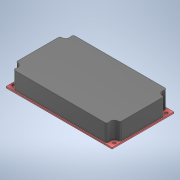
# Autodesk Inventor part: SUSTAINA-Core-Board
Saved by Autodesk Inventor 2022.3 (Build 263350000, 350)
## iProperties
Part Number: SUSTAINA-Core-Board
Material: 一般
Document SubType Name: Modeling
Designer: Masato Kubotera
Density: 1 g/cm^3
Appearance: 既定
Description: CircuitBoard
Author: Masato Kubotera
Autodesk Inventor part; units mm, degrees
ref_plane "YZ Plane" through (0, 0, 0) normal (1, 0, 0) x (0, 1, 0)
ref_plane "XZ Plane" through (0, 0, 0) normal (0, 1, 0) x (-1, 0, 0)
ref_plane "XY Plane" through (0, 0, 0) normal (0, 0, 1) x (1, 0, 0)
derived "Cockpit_circuit_board_frame.ipt"
sketch "スケッチ3" plane through (0, 0, -88.5) normal (0, 0, 1) x (1, 0, 0)
  line L0 (20.25, -135) -> (20.25, 0)
  line L1 (-83.25, 0) -> (-83.25, -135)
  line L2 (-31.5, -135) -> (-31.5, 0) construction
  line L3 (-83.25, -67.5) -> (20.25, -67.5) construction
  line L4 (-52.45, 1.4849) -> (-52.45, 5)
  line L5 (-52.45, 5) -> (-10.55, 5)
  line L6 (-10.55, 5) -> (-10.55, 1.4849)
  arc A0 (-53.9349, 0) -> (-52.45, 1.4849) centre (-53.1925, 0.7425) ccw
  arc A1 (-10.55, 1.4849) -> (-9.0651, 0) centre (-9.8075, 0.7425) ccw
  line L7 (-53.9349, 0) -> (-83.25, 0)
  line L8 (20.25, 0) -> (-9.0651, 0)
  line L9 (-10.55, 0) -> (-52.45, 0)
  line L10 (-10.55, -135) -> (-52.45, -135)
  arc A2 (-52.45, -136.4849) -> (-53.9349, -135) centre (-53.1925, -135.7425) ccw
  line L11 (-52.45, -136.4849) -> (-52.45, -140)
  line L12 (-52.45, -140) -> (-10.55, -140)
  line L13 (-10.55, -140) -> (-10.55, -136.4849)
  arc A3 (-9.0651, -135) -> (-10.55, -136.4849) centre (-9.8075, -135.7425) ccw
  line L14 (20.25, -135) -> (-9.0651, -135)
  line L15 (-53.9349, -135) -> (-83.25, -135)
  line L16 (18, -127.5) -> (-52, -127.5) construction
  line L17 (-52, -127.5) -> (-52, -7.5) construction
  line L18 (-52, -7.5) -> (18, -7.5) construction
  line L19 (18, -7.5) -> (18, -127.5) construction
  line L20 (18, -127.5) -> (-52, -7.5) construction
  line L21 (-52, -127.5) -> (18, -7.5) construction
  line L22 (-48.5, -116.5) -> (-48.5, -18.5)
  line L23 (-38.5627, -9.5) -> (4.5627, -9.5)
  line L24 (12.5, -10.5) -> (-46.5, -10.5) construction
  line L25 (-46.5, -10.5) -> (-46.5, -124.5) construction
  line L26 (-46.5, -124.5) -> (12.5, -124.5) construction
  line L27 (12.5, -124.5) -> (12.5, -10.5) construction
  line L28 (12.5, -10.5) -> (-46.5, -124.5) construction
  line L29 (-46.5, -10.5) -> (12.5, -124.5) construction
  circle A4 centre (12.5, -10.5) radius 2
  circle A5 centre (-46.5, -10.5) radius 2
  arc A6 (-46.5, -16.5) -> (-40.5471, -11.25) centre (-46.5, -10.5) ccw
  arc A7 (6.5471, -11.25) -> (12.5, -16.5) centre (12.5, -10.5) ccw
  line L30 (14.5, -18.5) -> (14.5, -116.5)
  line L31 (-17, -7.5) -> (-17, -127.5) construction
  line L32 (-76.25, -65) -> (-56.5, -65)
  line L33 (-54.5, -63) -> (-54.5, -7)
  line L34 (-56.5, -5) -> (-76.25, -5)
  line L35 (-78.25, -7) -> (-78.25, -63)
  arc A8 (-78.25, -63) -> (-76.25, -65) centre (-76.25, -63) ccw
  arc A9 (-56.5, -65) -> (-54.5, -63) centre (-56.5, -63) ccw
  arc A10 (-54.5, -7) -> (-56.5, -5) centre (-56.5, -7) ccw
  arc A11 (-76.25, -5) -> (-78.25, -7) centre (-76.25, -7) ccw
  arc A12 (-46.5, -16.5) -> (-48.5, -18.5) centre (-46.5, -18.5) ccw
  arc A13 (-38.5627, -9.5) -> (-40.5471, -11.25) centre (-38.5627, -11.5) ccw
  arc A14 (6.5471, -11.25) -> (4.5627, -9.5) centre (4.5627, -11.5) ccw
  arc A15 (14.5, -18.5) -> (12.5, -16.5) centre (12.5, -18.5) ccw
  line L36 (-54.5, -72) -> (-54.5, -128)
  line L37 (-78.25, -128) -> (-78.25, -72)
  arc A16 (-54.5, -72) -> (-56.5, -70) centre (-56.5, -72) ccw
  line L38 (-76.25, -70) -> (-56.5, -70)
  arc A17 (-76.25, -70) -> (-78.25, -72) centre (-76.25, -72) ccw
  line L39 (-56.5, -130) -> (-76.25, -130)
  arc A18 (-56.5, -130) -> (-54.5, -128) centre (-56.5, -128) ccw
  arc A19 (-78.25, -128) -> (-76.25, -130) centre (-76.25, -128) ccw
  arc A20 (-48.5, -116.5) -> (-46.5, -118.5) centre (-46.5, -116.5) ccw
  arc A21 (-40.5471, -123.75) -> (-46.5, -118.5) centre (-46.5, -124.5) ccw
  circle A22 centre (-46.5, -124.5) radius 2
  arc A23 (-40.5471, -123.75) -> (-38.5627, -125.5) centre (-38.5627, -123.5) ccw
  line L40 (-38.5627, -125.5) -> (4.5627, -125.5)
  arc A24 (4.5627, -125.5) -> (6.5471, -123.75) centre (4.5627, -123.5) ccw
  circle A25 centre (12.5, -124.5) radius 2
  arc A26 (12.5, -118.5) -> (6.5471, -123.75) centre (12.5, -124.5) ccw
  arc A27 (12.5, -118.5) -> (14.5, -116.5) centre (12.5, -116.5) ccw
  line L41 (12.5, -8.0316) -> (12.5, 3.8973)
  point P0 (0, 0)
  point P1 (-31.5, -67.5)
  point P2 (-17, -67.5)
  point P3 (-48.5, -16.1569)
  point P4 (-40.5839, -9.5)
  point P5 (6.5839, -9.5)
  point P6 (14.5, -16.1569)
ref_plane "作業平面1" through (20.25, 0, -88.5) normal (0, 0, -1) x (0, -1, 0)
sketch "スケッチ2" plane through (20.25, 0, -88.5) normal (0, 0, -1) x (0, -1, 0)
  line L0 (127.5, 72.25) -> (7.5, 72.25) projected
  line L1 (127.5, 2.25) -> (127.5, 72.25) projected
  line L2 (7.5, 72.25) -> (7.5, 2.25) projected
  line L3 (7.5, 2.25) -> (127.5, 2.25) projected
  circle A0 centre (10.5, 66.75) radius 2 projected
  circle A1 centre (10.5, 7.75) radius 2 projected
  circle A2 centre (124.5, 66.75) radius 2 projected
  circle A3 centre (124.5, 7.75) radius 2 projected
  circle A4 centre (10.5, 7.75) radius 1.6
  circle A5 centre (10.5, 66.75) radius 1.6
  circle A6 centre (124.5, 66.75) radius 1.6
  circle A7 centre (124.5, 7.75) radius 1.6
  arc A8 (120.3462, 68.4808) -> (124.5, 62.25) centre (124.5, 66.75) ccw
  line L4 (118.5, 71.25) -> (16.5, 71.25)
  line L5 (126.5, 60.25) -> (126.5, 14.25)
  line L6 (67.5, 103.5) -> (67.5, 0) construction
  line L7 (7.5, 37.25) -> (127.5, 37.25) construction
  arc A9 (10.5, 62.25) -> (14.6538, 68.4808) centre (10.5, 66.75) ccw
  arc A10 (124.5, 12.25) -> (120.3462, 6.0192) centre (124.5, 7.75) ccw
  arc A11 (14.6538, 6.0192) -> (10.5, 12.25) centre (10.5, 7.75) ccw
  line L8 (118.5, 3.25) -> (16.5, 3.25)
  line L9 (8.5, 14.25) -> (8.5, 60.25)
  arc A12 (120.3462, 68.4808) -> (118.5, 71.25) centre (118.5, 69.25) ccw
  arc A13 (126.5, 60.25) -> (124.5, 62.25) centre (124.5, 60.25) ccw
  arc A14 (124.5, 12.25) -> (126.5, 14.25) centre (124.5, 14.25) ccw
  arc A15 (118.5, 3.25) -> (120.3462, 6.0192) centre (118.5, 5.25) ccw
  arc A16 (14.6538, 6.0192) -> (16.5, 3.25) centre (16.5, 5.25) ccw
  arc A17 (8.5, 14.25) -> (10.5, 12.25) centre (10.5, 14.25) ccw
  arc A18 (10.5, 62.25) -> (8.5, 60.25) centre (10.5, 60.25) ccw
  arc A19 (16.5, 71.25) -> (14.6538, 68.4808) centre (16.5, 69.25) ccw
  point P0 (0, 20.25)
  point P1 (124.5, 71.25)
  point P2 (126.5, 62.7189)
  point P3 (10.5, 71.25)
  point P4 (126.5, 11.7811)
  point P5 (8.5, 62.7189)
  point P6 (124.5, 3.25)
  point P7 (10.5, 3.25)
  point P8 (8.5, 11.7811)
  dimension "d5" = 3.2
  dimension "d6" = 3.2
  dimension "d7" = 3.2
  dimension "d8" = 3.2
  dimension "d9" = 1
  dimension "d10" = 1
  dimension "d12" = 4.5
  dimension "d13" = 2
  constraints: 32 point on circle, 16 centre point, 16 tangent, 9 symmetric about line, 8 end point, 8 point on line, 7 equal radius, 5 coincident, 2 horizontal, 2 parallel, 3 other
  measures "d5" diameter of A4
  measures "d6" diameter of A5
  measures "d7" diameter of A6
  measures "d8" diameter of A7
  measures "d9" distance between parallel lines of L4 L0
  measures "d10" distance between parallel lines of L1 L5
  measures "d12" radius of A8
  measures "d13" radius of A12
extrude "押し出し1" add sketch "スケッチ2" against normal blind 1.6 contours L1 L3 L2 L0 | A0 | A1 | A2 | A3 | A8 A13 L5 A14 A10 A15 L8 A16 A11 A17 L9 A18 A9 A19 L4 A12
extrude "Extrusion2" add sketch "スケッチ2" against normal blind 21.1 contours A8 A13 L5 A14 A10 A15 L8 A16 A11 A17 L9 A18 A9 A19 L4 A12
equation "\"d6\" = d5"
equation "\"d7\" = d5"
equation "\"d8\" = d5"
equation "\"d10\" = d9"
